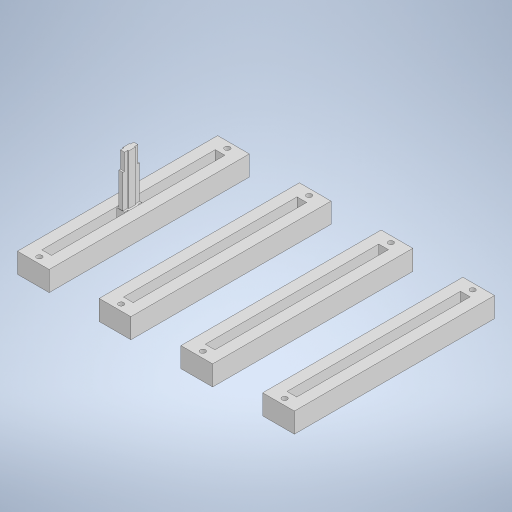
# Autodesk Inventor part: noise-synth-enclosure
Saved by Autodesk Inventor 2024.1 (Build 281209000, 209)
## iProperties
Created: 2025-09-17
Part Number: noise-synth-enclosure
Material: Generic
Document SubType Name: Modeling
Designer: iwheard
Density: 1 g/cm^3
Appearance: Default
Author: iwheard
Autodesk Inventor part; units mm, degrees
ref_plane "YZ Plane" through (0, 0, 0) normal (1, 0, 0) x (0, 1, 0)
ref_plane "XZ Plane" through (0, 0, 0) normal (0, 1, 0) x (-1, 0, 0)
ref_plane "XY Plane" through (0, 0, 0) normal (0, 0, 1) x (1, 0, 0)
sketch "Sketch1" plane through (0, 0, 0) normal (0, 1, 0) x (-1, 0, 0)
  line L0 (0, 0) -> (-9.5, 0)
  line L1 (-9.5, 0) -> (-9.5, -60)
  line L2 (-9.5, -60) -> (0, -60)
  line L3 (0, -60) -> (0, 0)
  line L4 (-24.5, 0) -> (-34, 0)
  line L5 (-34, 0) -> (-34, -60)
  line L6 (-34, -60) -> (-24.5, -60)
  line L7 (-24.5, -60) -> (-24.5, 0)
  line L8 (-49, 0) -> (-58.5, 0)
  line L9 (-58.5, 0) -> (-58.5, -60)
  line L10 (-58.5, -60) -> (-49, -60)
  line L11 (-49, -60) -> (-49, 0)
  line L12 (-83, 0) -> (-73.5, 0)
  line L13 (-73.5, 0) -> (-73.5, -60)
  line L14 (-73.5, -60) -> (-83, -60)
  line L15 (-83, -60) -> (-83, 0)
  dimension "d0" = 60
  dimension "d1" = 9.5
  dimension "d2" = 9.5
  dimension "d3" = 9.5
  dimension "d4" = 9.5
  dimension "d5" = 15
  dimension "d6" = 15
  dimension "d7" = 15
  constraints: 32 end point, 6 horizontal alignment, 1 coincident, 1 horizontal
  measures "d0" distance between parallel lines of L2 L0
  measures "d1" distance between parallel lines of L1 L3
  measures "d2" distance between parallel lines of L5 L7
  measures "d3" distance between parallel lines of L9 L11
  measures "d4" distance between parallel lines of L15 L13
  measures "d5" distance between parallel lines of L7 L1
  measures "d6" distance between parallel lines of L11 L5
  measures "d7" distance between parallel lines of L13 L9
extrude "Extrusion1" add sketch "Sketch1" against normal blind 6
sketch "Sketch2" plane through (0, 0, 0) normal (0, 1, 0) x (1, 0, 0)
  line L0 (3.3, 4) -> (6.2, 4)
  line L1 (6.2, 4) -> (6.2, 56)
  line L2 (6.2, 56) -> (3.3, 56)
  line L3 (3.3, 56) -> (3.3, 4)
  line L4 (0, 60) -> (0, 0) projected
  line L5 (9.5, 0) -> (9.5, 60) projected
  line L6 (0, 0) -> (9.5, 0) projected
  line L7 (9.5, 60) -> (0, 60) projected
  line L8 (27.8, 4) -> (30.7, 4)
  line L9 (30.7, 4) -> (30.7, 56)
  line L10 (30.7, 56) -> (27.8, 56)
  line L11 (27.8, 56) -> (27.8, 4)
  line L12 (52.3, 4) -> (55.2, 4)
  line L13 (55.2, 4) -> (55.2, 56)
  line L14 (55.2, 56) -> (52.3, 56)
  line L15 (52.3, 56) -> (52.3, 4)
  line L16 (76.8, 4) -> (79.7, 4)
  line L17 (79.7, 4) -> (79.7, 56)
  line L18 (79.7, 56) -> (76.8, 56)
  line L19 (76.8, 56) -> (76.8, 4)
  line L20 (24.5, 60) -> (24.5, 0) projected
  line L21 (34, 0) -> (34, 60) projected
  line L22 (49, 60) -> (49, 0) projected
  line L23 (58.5, 0) -> (58.5, 60) projected
  line L24 (73.5, 60) -> (73.5, 0) projected
  line L25 (83, 0) -> (83, 60) projected
  point P0 (4.75, 56)
  point P1 (29.25, 56)
  point P2 (53.75, 56)
  point P3 (78.25, 56)
  point P4 (4.75, 4)
  point P5 (29.25, 4)
  point P6 (53.75, 4)
  point P7 (78.25, 4)
  dimension "d10" = 3.3
  dimension "d11" = 3.3
  dimension "d12" = 4
  dimension "d13" = 4
  dimension "d14" = 3.3
  dimension "d15" = 3.3
  dimension "d16" = 3.3
  dimension "d17" = 3.3
  dimension "d18" = 3.3
  dimension "d19" = 3.3
  constraints: 32 end point, 8 midpoint, 6 horizontal alignment
  measures "d10" distance between parallel lines of L4 L3
  measures "d11" distance between parallel lines of L5 L1
  measures "d12" distance between parallel lines of L6 L0
  measures "d13" distance between parallel lines of L7 L2
  measures "d14" distance between parallel lines of L20 L11
  measures "d15" distance between parallel lines of L21 L9
  measures "d16" distance between parallel lines of L22 L15
  measures "d17" distance between parallel lines of L23 L13
  measures "d18" distance between parallel lines of L24 L19
  measures "d19" distance between parallel lines of L25 L17
extrude "Extrusion2" cut sketch "Sketch2" against normal blind 4.3 contours L3 L2 L1 L0 | L11 L10 L9 L8 | L15 L14 L13 L12 | L19 L18 L17 L16
sketch "Sketch3" plane through (0, 0, 0) normal (0, 1, 0) x (1, 0, 0)
  line L0 (3.87, 27.759) -> (5.63, 27.759)
  line L1 (5.63, 27.759) -> (5.63, 29.729)
  line L2 (5.63, 29.729) -> (3.87, 29.729)
  line L3 (3.87, 29.729) -> (3.87, 27.759)
  line L4 (3.3, 4) -> (3.3, 56) projected
  line L5 (6.2, 56) -> (6.2, 4) projected
  line L6 (4.14, 26.264) -> (5.36, 26.264)
  line L7 (5.36, 26.264) -> (5.36, 31.224)
  line L8 (5.36, 31.224) -> (4.14, 31.224)
  line L9 (4.14, 31.224) -> (4.14, 26.264)
  point P0 (0, 0)
  point P1 (4.14, 27.759)
  point P2 (5.36, 27.759)
  point P3 (5.36, 29.729)
  point P4 (4.14, 29.729)
  dimension "d22" = 1.76
  dimension "d24" = 2.9
  dimension "d25" = 0.57
  dimension "d26" = 1.97
  dimension "d27" = 4.96
  dimension "d28" = 1.495
  dimension "d29" = 1.22
  dimension "d30" = 0.27
  constraints: 16 end point
  measures "d22" distance between parallel lines of L1 L3
  measures "d24" distance between parallel lines of L5 L4
  measures "d25" distance between parallel lines of L4 L3
  measures "d26" distance between parallel lines of L2 L0
  measures "d27" distance between parallel lines of L8 L6
  measures "d28" distance between parallel lines of L0 L6
  measures "d29" distance between parallel lines of L7 L9
  measures "d30" distance between parallel lines of L3 L9
extrude "Extrusion3" add sketch "Sketch3" along normal blind 15
sketch "Sketch4" plane through (0, 15, 0) normal (0, 1, 0) x (1, 0, 0)
  line L0 (3.87, 27.759) -> (4.14, 27.759) projected
  line L1 (4.14, 27.759) -> (4.14, 26.264) projected
  line L2 (4.14, 26.264) -> (5.36, 26.264) projected
  line L3 (5.36, 26.264) -> (5.36, 27.759) projected
  line L4 (5.36, 27.759) -> (5.63, 27.759) projected
  line L5 (5.63, 27.759) -> (5.63, 29.729) projected
  line L6 (5.63, 29.729) -> (5.36, 29.729) projected
  line L7 (5.36, 29.729) -> (5.36, 31.224) projected
  line L8 (5.36, 31.224) -> (4.14, 31.224) projected
  line L9 (4.14, 31.224) -> (4.14, 29.729) projected
  line L10 (4.14, 29.729) -> (3.87, 29.729) projected
  line L11 (3.87, 29.729) -> (3.87, 27.759) projected
  line L12 (5.36, 26.754) -> (4.14, 26.754)
  line L13 (4.14, 30.734) -> (5.36, 30.734)
  point P0 (0, 0)
  dimension "d33" = 3.98
  dimension "d34" = 4.96
  dimension "d35" = 0.49
  constraints: 4 end point, 4 point on line
  measures "d33" distance between parallel lines of L13 L12
  measures "d34" distance between parallel lines of L8 L2
  measures "d35" distance between parallel lines of L2 L12
extrude "Extrusion4" cut sketch "Sketch4" against normal blind 5 contours L12 L3 L2 L1 | L9 L8 L7 L13
sketch "Sketch5" plane through (0, 0, 0) normal (0, -1, 0) x (1, 0, 0)
  line L0 (4.14, -30.734) -> (4.14, -31.224) projected
  line L1 (5.36, -30.734) -> (4.14, -30.734) projected
  line L2 (5.36, -31.224) -> (5.36, -30.734) projected
  line L3 (4.14, -31.224) -> (5.36, -31.224) projected
  line L4 (4.14, -26.754) -> (5.36, -26.754) projected
  line L5 (5.36, -26.754) -> (5.36, -27.759) projected
  line L6 (5.36, -27.759) -> (5.63, -27.759) projected
  line L7 (5.63, -27.759) -> (5.63, -29.729) projected
  line L8 (5.63, -29.729) -> (5.36, -29.729) projected
  line L9 (5.36, -29.729) -> (5.36, -30.734) projected
  line L10 (5.36, -30.734) -> (4.14, -30.734) projected
  line L11 (4.14, -30.734) -> (4.14, -29.729) projected
  line L12 (4.14, -29.729) -> (3.87, -29.729) projected
  line L13 (3.87, -29.729) -> (3.87, -27.759) projected
  line L14 (3.87, -27.759) -> (4.14, -27.759) projected
  line L15 (4.14, -27.759) -> (4.14, -26.754) projected
  line L16 (5.36, -26.754) -> (5.36, -26.264) projected
  line L17 (4.14, -26.754) -> (5.36, -26.754) projected
  line L18 (4.14, -26.264) -> (4.14, -26.754) projected
  line L19 (5.36, -26.264) -> (4.14, -26.264) projected
  line L20 (3.3, -27.189) -> (3.3, -30.299)
  line L21 (3.3, -30.299) -> (3.57, -30.299)
  line L22 (3.57, -30.299) -> (3.57, -31.304)
  line L23 (3.57, -31.304) -> (5.93, -31.304)
  line L24 (5.93, -31.304) -> (5.93, -30.299)
  line L25 (5.93, -30.299) -> (6.2, -30.299)
  line L26 (6.2, -30.299) -> (6.2, -27.189)
  line L27 (6.2, -27.189) -> (5.93, -27.189)
  line L28 (5.93, -27.189) -> (5.93, -26.184)
  line L29 (5.93, -26.184) -> (3.57, -26.184)
  line L30 (3.57, -26.184) -> (3.57, -27.189)
  line L31 (3.57, -27.189) -> (3.3, -27.189)
  line L32 (3.3, -4) -> (3.3, -56) projected
  point P0 (0, 0)
  constraints: 24 end point, 1 point on line, 11 other
extrude "Extrusion5" add sketch "Sketch5" along normal up to surface (4.3 mm away) separate body
sketch "Sketch6" plane through (0, 0, 0) normal (0, 1, 0) x (1, 0, 0)
  circle A0 centre (4.75, 58.175) radius 0.8
  circle A1 centre (29.25, 58.175) radius 0.8
  circle A2 centre (53.75, 58.175) radius 0.8
  circle A3 centre (78.25, 58.175) radius 0.8
  circle A4 centre (4.75, 1.825) radius 0.8
  circle A5 centre (29.25, 1.825) radius 0.8
  circle A6 centre (53.75, 1.825) radius 0.8
  circle A7 centre (78.25, 1.825) radius 0.8
  line L0 (9.5, 60) -> (0, 60) projected
  line L1 (0, 0) -> (9.5, 0) projected
  line L2 (34, 60) -> (24.5, 60) projected
  line L3 (24.5, 0) -> (34, 0) projected
  line L4 (58.5, 60) -> (49, 60) projected
  line L5 (83, 60) -> (73.5, 60) projected
  line L6 (73.5, 0) -> (83, 0) projected
  point P0 (4.75, 60)
  point P1 (29.25, 60)
  point P2 (4.75, 0)
  point P3 (29.25, 0)
  point P4 (53.75, 60)
  point P5 (53.75, 60)
  point P6 (78.25, 60)
  point P7 (78.25, 0)
  dimension "d40" = 1.6
  dimension "d41" = 1.825
  dimension "d42" = 56.35
  dimension "d43" = 1.825
  constraints: 8 centre point, 8 midpoint, 8 vertical alignment, 7 equal radius, 6 horizontal alignment
  measures "d40" diameter of A0
  measures "d41" distance from line of A0.centre L0
  measures "d42" distance of A4.centre A0.centre
  measures "d43" distance from line of L1 A4.centre
extrude "Extrusion6" cut sketch "Sketch6" against normal blind 5 bodies 1
equation "\"d2\" = d1"
equation "\"d3\" = d2"
equation "\"d4\" = d3"
equation "\"d6\" = d5"
equation "\"d7\" = d6"
equation "\"d11\" = d10"
equation "\"d13\" = d12"
equation "\"d25\" = -0.5 * d22 + 0.5 * d24"
equation "\"d28\" = -0.5 * d26 + 0.5 * d27"
equation "\"d30\" = -0.5 * d29 + 0.5 * d22"
equation "\"d35\" = -0.5 * d33 + 0.5 * d34"
body "Solid1"
body "Solid2"
